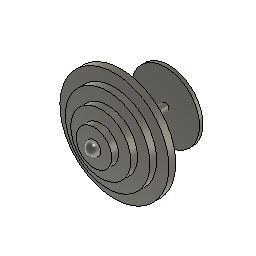
Doorknobs_final_additive (Autodesk Fusion 360 design; units mm, degrees)
Autodesk Fusion 360 part; units mm, degrees
note: some values were not read from the file. Set by a fixed rule: which sketch regions a step uses.
sketch "Sketch1" plane through (0, 0, 0) normal (1, 0, 0) x (0, 1, 0) in component "Doorknob_Revolve_Addition"
  line L0 (0, 0) -> (0, 31.75)
  line L1 (-25.4, 3.175) -> (-25.4, 16.51)
  line L2 (-31.75, 16.51) -> (-31.75, 27.94)
  line L3 (-31.75, 27.94) -> (-38.1, 27.94)
  line L4 (-38.1, 27.94) -> (-38.1, 39.37)
  line L5 (-25.4, 16.51) -> (-31.75, 16.51)
  line L6 (-38.1, 39.37) -> (-44.45, 39.37)
  line L7 (-44.45, 39.37) -> (-44.45, 50.8)
  line L8 (-44.45, 50.8) -> (-50.8, 50.8)
  line L9 (-50.8, 50.8) -> (-50.8, 39.37)
  line L10 (-50.8, 39.37) -> (-57.15, 39.37)
  line L11 (-57.15, 39.37) -> (-57.15, 27.94)
  line L12 (-57.15, 27.94) -> (-63.5, 27.94)
  line L13 (-63.5, 27.94) -> (-63.5, 16.51)
  line L14 (-63.5, 16.51) -> (-69.85, 16.51)
  line L15 (-69.85, 16.51) -> (-69.85, 6.35)
  line L16 (-76.2, 0) -> (0, 0)
  arc A0 (-69.85, 6.35) -> (-76.2, 0) centre (-69.85, 0) ccw
  line L17 (0, 31.75) -> (-3.175, 31.75)
  line L18 (-3.175, 31.75) -> (-3.175, 3.175)
  line L19 (-3.175, 3.175) -> (-25.4, 3.175)
  dimension "d4" = 76.2
  dimension "d5" = 31.75
  dimension "d6" = 50.8
  dimension "d10" = 11.43
  dimension "d11" = 11.43
  dimension "d12" = 11.43
  dimension "d13" = 6.35
  dimension "d14" = 6.35
  dimension "d15" = 6.35
  dimension "d16" = 6.35
  dimension "d20" = 6.35
  dimension "d22" = 3.175
  dimension "d23" = 3.175
  dimension "d24" = 22.225
  constraint coincident L0.start L16.end
  constraint vertical L0
  constraint parallel L0 L2
  constraint perpendicular L0 L3
  constraint perpendicular L3 L4
  constraint perpendicular L1 L5
  constraint perpendicular L4 L6
  constraint perpendicular L6 L7
  constraint perpendicular L7 L8
  constraint perpendicular L8 L9
  constraint perpendicular L9 L10
  constraint perpendicular L10 L11
  constraint perpendicular L9 L12
  constraint perpendicular L12 L13
  constraint perpendicular L9 L14
  constraint perpendicular L14 L15
  constraint horizontal L16
  constraint collinear L5 L14
  constraint collinear L3 L12
  constraint collinear L6 L10
  constraint equal L5 L14
  constraint equal L3 L12
  constraint equal L6 L10
  constraint coincident L16 A0.centre
  constraint perpendicular L0 L17
  constraint vertical L18
  constraint horizontal L19
  measures "d4" distance of L0.start L16.start
  measures "d5" distance of L0.start L0.end
  measures "d6" distance of L8 L16
  measures "d10" distance of L6 L8
  measures "d11" distance of L3.end L4.end
  measures "d12" distance of L2.start L2.end
  measures "d13" distance of L7.end L8.end
  measures "d14" distance of L4.end L6.end
  measures "d15" distance of L2.end L3.end
  measures "d16" distance of L1.end L2.start
  measures "d20" radius of A0
  measures "d22" distance of L0.end L17.end
  measures "d23" distance of L16 L19
  measures "d24" distance of L1 L18
revolve "Revolve1" add sketch "Sketch1" angle 360 about axis through (0, -76.2, 0) along (0, 1, 0) in component "Doorknob_Revolve_Addition"
component "Doorknob_Revolve_Addition" placed x (1, 0, 0) y (0, 1, 0) z (0, 0, 1) at (0, 0, 0)
equation "d5 = ( 2.5 / 2 ) * 1 in"
equation "d11 = d10"
equation "d12 = d10"
equation "d14 = d13"
equation "d15 = d14"
equation "d16 = d13"
